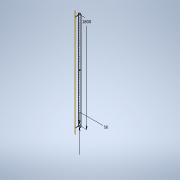
# Autodesk Inventor part: armj3
Saved by Autodesk Inventor 2020 (Build 240168000, 168)
## iProperties
Created: 2020-07-11
Part Number: armj3
Material: Aluminum 6061
Document SubType Name: Modeling
Designer: Vikki
Density: 2.7 g/cm^3
Appearance: Glossy - Black
Mass: 33.9292 g
Surface Area: 53.4071 cm^2
Volume: 12.5664 cm^3
Author: Vikki
Autodesk Inventor part; units mm, degrees
ref_plane "YZ Plane" through (0, 0, 0) normal (1, 0, 0) x (0, 1, 0)
ref_plane "XZ Plane" through (0, 0, 0) normal (0, 1, 0) x (-1, 0, 0)
sketch "Sketch1" plane through (0, 0, 0) normal (0, 0, 1) x (1, 0, 0)
  line L0 (0, 0) -> (0, -1800) construction
  line L1 (-25, 0) -> (-25, -1800)
  line L2 (25, -1800) -> (25, 0)
  arc A0 (25, 0) -> (-25, 0) centre (0, 0) ccw
  arc A1 (-25, -1800) -> (25, -1800) centre (0, -1800) ccw
  point P0 (0, -900)
  dimension "d0" = 50
  dimension "d1" = 1800
  constraints: 8 end point, 4 point on circle, 4 tangent, 2 centre point, 1 midpoint, 1 parallel, 1 vertical
  measures "d0" diameter of A1
  measures "d1" distance of L0.start L0.end
ref_plane "Work Plane1" through (0, 0, 80) normal (0, 0, 1) x (1, 0, 0)
sketch "Sketch2" plane through (0, 0, 80) normal (0, 0, 1) x (1, 0, 0)
  line L0 (-25, 0) -> (-25, -1800) projected
  arc A0 (25, 0) -> (-25, 0) centre (0, 0) ccw projected
  line L1 (25, -1800) -> (25, 0) projected
  arc A1 (-25, -1800) -> (25, -1800) centre (0, -1800) ccw projected
  circle A2 centre (0, 0) radius 5
  circle A3 centre (0, -1800) radius 5
  dimension "d3" = 10
  dimension "d4" = 10
  constraints: 2 centre point, 2 coincident
  measures "d3" diameter of A2
  measures "d4" diameter of A3
extrude "Extrusion1" add sketch "Sketch2" against normal up to surface (80 mm away) contours A2 | A3
body "Solid1"
